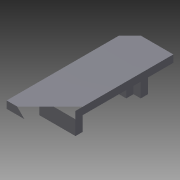
# Autodesk Inventor part: track
Saved by Autodesk Inventor 2016 (Build 200138000, 138)
## iProperties
Created: 2011-12-02
Part Number: track
Material: Rubber
Document SubType Name: Modeling
Designer: caparks
Mass: 3454.19 g
Surface Area: 841.127 cm^2
Volume: 430.16 cm^3
Density: 0.93 g/cm^3
Appearance: Rubber - Black
Author: caparks
Keywords: =<Description>  <Part Number>
Autodesk Inventor part; units mm, degrees
ref_plane "YZ Plane" through (0, 0, 0) normal (1, 0, 0) x (0, 1, 0)
ref_plane "XZ Plane" through (0, 0, 0) normal (0, 1, 0) x (-1, 0, 0)
ref_plane "XY Plane" through (0, 0, 0) normal (0, 0, 1) x (1, 0, 0)
sketch "Sketch1" plane through (0, 0, 0) normal (0, 0, 1) x (1, 0, 0)
  line L0 (3, 1) -> (3, 0)
  line L1 (3, 0) -> (-3, 0)
  line L2 (-3, 0) -> (-3, 1)
  line L3 (3, 1) -> (-3, 1)
  point P0 (0, 0)
  point P1 (0, 0)
  dimension "d0" = 6
  dimension "d6" = 1
  constraints: 8 end point, 2 parallel, 1 coincident, 1 horizontal, 1 midpoint, 1 perpendicular
  measures "d0" distance of L0.end L1.end
  measures "d6" distance of L1.end L2.end
extrude "Extrusion1" add sketch "Sketch1" along normal mid plane 17
sketch "Sketch2" plane through (-3, 0, 8.5) normal (0, -1, 0) x (1, 0, 0)
  line L0 (0, -5.5) -> (5, -5.5)
  line L1 (5, -5.5) -> (5, -4.5)
  line L2 (1, -4.5) -> (0, -4.5)
  line L3 (0, -4.5) -> (0, -5.5)
  line L4 (6, -3.5) -> (1, -3.5)
  line L5 (1, -3.5) -> (1, -4.5)
  line L6 (5, -4.5) -> (6, -4.5)
  line L7 (6, -4.5) -> (6, -3.5)
  line L8 (0, -17) -> (0, 0) projected
  line L9 (6, 0) -> (6, -17) projected
  line L10 (6, 0) -> (0, 0) projected
  line L11 (6, 0) -> (0, 0) projected
  line L12 (0, -17) -> (0, 0) projected
  line L13 (0, -17) -> (6, -17) projected
  line L14 (6, 0) -> (6, -17) projected
  line L15 (-1.2, -8.5) -> (7.2, -8.5) projected
  line L16 (5, -11.5) -> (5, -12.5)
  line L17 (1, -12.5) -> (0, -12.5)
  line L18 (0, -12.5) -> (0, -11.5)
  line L19 (6, -13.5) -> (1, -13.5)
  line L20 (1, -13.5) -> (1, -12.5)
  line L21 (5, -12.5) -> (6, -12.5)
  line L22 (6, -12.5) -> (6, -13.5)
  line L23 (0, -11.5) -> (5, -11.5)
  point P0 (3, -8.5)
  dimension "d7" = 1
  dimension "d8" = 1
  dimension "d9" = 2
  dimension "d10" = 3.5
  constraints: 32 end point, 8 symmetric about line, 4 parallel, 2 collinear, 2 equal length, 2 horizontal, 2 perpendicular
  measures "d7" distance of L2.end L0.start
  measures "d8" distance of L2.start L2.end
  measures "d9" distance between parallel lines of L4 L0
  measures "d10" distance between parallel lines of L10 L4
extrude "Extrusion2" add sketch "Sketch2" along normal blind 2 contours L3 L2 L5 L4 L7 L6 L1 L0 | L23 L16 L21 L9 L19 L20 L17 L8
sketch "Sketch3" plane through (-3, 0, 3) normal (0, -1, 0) x (1, 0, 0)
  line L0 (6, 1) -> (5, 1) projected
  line L1 (5, 1) -> (5, 0) projected
  line L2 (5, 0) -> (0, 0) projected
  line L3 (0, -6) -> (0, 0) projected
  line L4 (0, -6) -> (5, -6) projected
  line L5 (5, -6) -> (5, -7) projected
  line L6 (5, -7) -> (6, -7) projected
  line L7 (6, 1) -> (6, -7) projected
  line L8 (4, -1.5) -> (0, -1.5)
  line L9 (0, -1.5) -> (0, -4.5)
  line L10 (0, -4.5) -> (4, -4.5)
  line L11 (4, -4.5) -> (4, -1.5)
  line L12 (0, -6) -> (0, 0) projected
  line L13 (-1.2, -3) -> (7.2, -3) projected
  point P0 (3, -3)
  point P1 (0, -3)
  dimension "d13" = 4
  dimension "d14" = 3
  constraints: 8 end point, 2 midpoint, 2 parallel, 1 horizontal, 1 perpendicular, 1 other
  measures "d13" distance of L9.end L10.end
  measures "d14" distance of L10.end L8.start
extrude "Extrusion3" cut sketch "Sketch3" against normal through all contours L13 L3 L8 L11 | L11 L10 L3 L13
sketch "Sketch4" plane through (-3, 1, 8.5) normal (0, 1, 0) x (1, 0, 0)
  line L0 (6, 2) -> (4, 2)
  line L1 (4, 2) -> (4, 15)
  line L2 (4, 15) -> (6, 15)
  line L3 (6, 15) -> (6, 2)
  line L4 (-1.2, 8.5) -> (7.2, 8.5) projected
  line L5 (6, 17) -> (6, 0) projected
  line L6 (4, 10) -> (4, 7) projected
  point P0 (3, 8.5)
  dimension "d17" = 13
  constraints: 8 end point, 2 collinear, 2 parallel, 1 horizontal, 1 perpendicular, 1 other
  measures "d17" distance of L0.end L1.end
extrude "Extrusion4" add sketch "Sketch4" along normal blind 2
body "Solid1"
